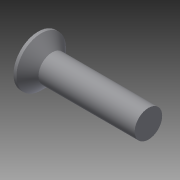
# Autodesk Inventor part: 零件4-4.1
Saved by Autodesk Inventor 2014 (Build 180170000, 170)
## iProperties
Created: 2018-10-26
Part Number: 零件4-4.1
Material: 常规
Document SubType Name: Modeling
Designer: Administrator
Density: 1 g/cm^3
Appearance: 默认
Author: Administrator
Autodesk Inventor part; units mm, degrees
ref_plane "YZ Plane" through (0, 0, 0) normal (1, 0, 0) x (0, 1, 0)
ref_plane "XZ Plane" through (0, 0, 0) normal (0, 1, 0) x (-1, 0, 0)
ref_plane "XY Plane" through (0, 0, 0) normal (0, 0, 1) x (1, 0, 0)
sketch "草图1" plane through (0, 0, 0) normal (0, 0, 1) x (1, 0, 0)
  line L0 (-25.3411, -1.0603) -> (77.0972, -1.0603)
  line L1 (71.6658, -1.0603) -> (71.6658, 8.9397)
  line L2 (71.6658, 8.9397) -> (1.6658, 8.9397)
  line L3 (1.6658, 8.9397) -> (-6.3342, 16.9397)
  line L4 (-6.3342, 16.9397) -> (-6.3342, -1.0603)
  line L5 (-6.3342, 16.9397) -> (-8.5111, 16.9397)
  line L6 (-8.5111, 16.9397) -> (-8.5111, -1.0603)
  line L7 (1.6658, 8.9397) -> (1.6658, -1.0603)
  arc A0 (-8.5111, 16.9397) -> (-13.3342, -1.0603) centre (22.6658, -1.0603) ccw
  line L8 (1.6658, 8.9397) -> (1.6658, 23.5751) construction
  point P0 (0, 0)
  dimension "d0" = 45
  dimension "d1" = 70
  dimension "d2" = 85
  dimension "d3" = 10
  dimension "d4" = 18
  dimension "d5" = 36
  constraints: 18 end point, 6 perpendicular, 6 point on line, 2 point on circle, 1 centre point, 1 collinear, 1 horizontal
  measures "d0" angle of L8 L3
  measures "d1" distance of L1.end L2.end
  measures "d2" distance of L1.start A0.end
  measures "d3" distance of L1.start L1.end
  measures "d4" distance of L3.end L4.end
  measures "d5" radius of A0
revolve "旋转1" add sketch "草图1" angle 360 about axis through (-25.3411, -1.0603, 0) along (1, 0, 0)
